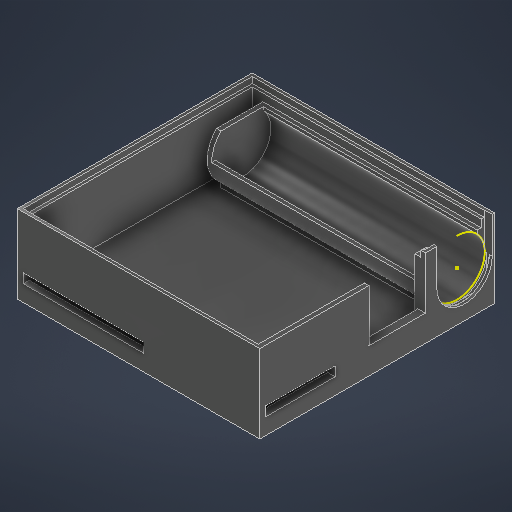
# Autodesk Inventor part: pudelko
Saved by Autodesk Inventor 2026.1 (Build 301233020, 233B)
## iProperties
Created: 2025-08-19
Part Number: pudelko
Material: Generic
Document SubType Name: Modeling
Designer: Paweł
Density: 1 g/cm^3
Appearance: Dark Gray
Mass: 30.7875 g
Surface Area: 279.129 cm^2
Volume: 30.7875 cm^3
Author: Paweł
Autodesk Inventor part; units mm, degrees
ref_plane "YZ Plane" through (0, 0, 0) normal (1, 0, 0) x (0, 1, 0)
ref_plane "XZ Plane" through (0, 0, 0) normal (0, 1, 0) x (-1, 0, 0)
ref_plane "XY Plane" through (0, 0, 0) normal (0, 0, 1) x (1, 0, 0)
sketch "Sketch1" plane through (0, 0, 0) normal (0, 1, 0) x (-1, 0, 0)
  line L0 (77.0121, 67.7143) -> (-2.9879, 67.7143)
  line L1 (-2.9879, 67.7143) -> (-2.9879, -12.2857)
  line L2 (-2.9879, -12.2857) -> (77.0121, -12.2857)
  line L3 (77.0121, -12.2857) -> (77.0121, 67.7143)
  point P0 (0, 0)
  dimension "d0" = 80
  dimension "d1" = 80
  constraints: 8 end point, 2 parallel, 1 horizontal, 1 perpendicular
  measures "d0" distance of L2.end L1.end
  measures "d1" distance of L0.end L1.end
extrude "Extrusion1" add sketch "Sketch1" along normal blind 2
sketch "Sketch2" plane through (0, 2, 0) normal (0, 1, 0) x (1, 0, 0)
  line L0 (2.9879, -67.7143) -> (2.9879, 12.2857) projected
  line L1 (2.9879, 12.2857) -> (-77.0121, 12.2857) projected
  line L2 (-77.0121, 12.2857) -> (-77.0121, -67.7143) projected
  line L3 (-77.0121, -67.7143) -> (2.9879, -67.7143) projected
  line L4 (0.9879, -65.7143) -> (0.9879, 10.2857)
  line L5 (0.9879, 10.2857) -> (-75.0121, 10.2857)
  line L6 (-75.0121, 10.2857) -> (-75.0121, -65.7143)
  line L7 (-75.0121, -65.7143) -> (0.9879, -65.7143)
  point P0 (0, 0)
  dimension "d4" = 2
  constraints: 8 end point, 3 other
  measures "d4" distance between parallel lines of L3 L7
extrude "Extrusion2" add sketch "Sketch2" along normal blind 20
sketch "Sketch4" plane through (-77.0121, 0, 67.7143) normal (0, 0, 1) x (1, 0, 0)
  line L0 (2, 2) -> (2, 22) projected
  line L1 (78, 2) -> (78, 22) projected
  line L2 (2, 12) -> (78, 12)
  line L3 (78, 12) -> (78, 2)
  line L4 (78, 2) -> (2, 2)
  line L5 (2, 2) -> (2, 12)
  line L6 (2, 2) -> (78, 2)
  line L7 (78, 2) -> (78, 7)
  line L8 (78, 7) -> (2, 7)
  line L9 (2, 7) -> (2, 2)
  line L10 (78, 2) -> (62, 2)
  line L11 (62, 2) -> (2, 2)
  line L12 (2, 2) -> (78, 2) projected
  line L13 (2, 2) -> (62, 2)
  line L14 (2, 3.4) -> (78, 3.4)
  line L15 (2, 6.5) -> (78, 6.5)
  line L16 (42, 2) -> (42, 7)
  point P0 (77.0121, 0)
  point P1 (2, 3.4)
  point P2 (42, 3.4)
  point P3 (42, 6.5)
  dimension "d53" = 16
  dimension "d54" = 1.4
  dimension "d55" = 0.5
  dimension "d130" = 40
  constraints: 28 end point, 7 point on line, 5 parallel, 3 perpendicular, 2 collinear, 2 horizontal, 2 midpoint
  measures "d53" distance of L6.end L10.end
  measures "d54" distance between parallel lines of L4 L14
  measures "d55" distance between parallel lines of L8 L15
  measures "d130" distance from line of L14.start L16
extrude "Extrusion4" cut sketch "Sketch4" against normal blind 20 contours L0 L15 L16 L14
sketch "Sketch5" plane through (0.9879, 2, -10.2857) normal (-1, 0, 0) x (0, 0, 1)
  line L0 (76, 0) -> (0, 0) projected
  line L1 (0, 0) -> (0, 20) projected
  circle A0 centre (10, 10) radius 9
  circle A1 centre (10, 10) radius 10
  circle A2 centre (10, 10) radius 10.5
  circle A3 centre (10, 10) radius 9.2
  line L2 (0, 20) -> (76, 20) projected
  line L3 (0, 10) -> (20.5, 10)
  line L4 (13.2016, 0) -> (16.2016, 0)
  line L5 (16.2016, 0) -> (16.2016, 1.5271)
  line L6 (10, 10) -> (10, 20)
  point P0 (10.2857, -2)
  point P1 (78, 0)
  point P2 (10, 0)
  point P3 (13.2016, 0)
  point P4 (13.2016, 20)
  point P5 (6.7984, 20)
  point P6 (0, 13.2016)
  point P7 (0.8, 10)
  point P8 (0, 10)
  point P9 (19.2, 10)
  point P10 (6.7984, 0)
  point P11 (0, 6.7984)
  point P12 (10, 19.2)
  dimension "d11" = 18
  dimension "d12" = 1
  dimension "d13" = 0.5
  dimension "d14" = 0.2
  dimension "d31" = 3
  constraints: 8 end point, 5 point on circle, 4 centre point, 4 midpoint, 4 point on line, 1 horizontal alignment, 1 parallel, 1 perpendicular
  measures "d11" diameter of A0
  measures "d12" radial gap between concentric circles of A0 A1
  measures "d13" radial gap between concentric circles of A1 A2
  measures "d14" radial gap between concentric circles of A0 A3
  measures "d31" distance of L4.start L4.end
extrude "Extrusion5" add sketch "Sketch5" along normal blind 71 contours L0 A2 L5 | L0 A1 L3 A2 | L0 A2 L1 A1 | A1 L3 A3 | L0 L1 A2 | L1 A2 L2 A1 | A1 L6 A3 L3 | L1 L2 A2 picked at (0.4271, 11.4241)
sketch "Sketch10" plane through (0, 2, 0) normal (0, 1, 0) x (1, 0, 0)
  line L0 (-70.0121, -2.9159) -> (-70.0121, -10.2143) projected
  line L1 (-70.0121, 10.2857) -> (-75.0121, 10.2857) projected
  line L2 (-70.0121, -10.2143) -> (-71.5121, -10.2143)
  line L3 (-71.5121, -10.2143) -> (-71.5121, 10.2857)
  line L4 (-71.5121, 10.2857) -> (-70.0121, 10.2857)
  line L5 (-70.0121, 10.2857) -> (-70.0121, -10.2143)
  point P0 (0, 0)
  point P1 (-70.0121, -5.9159)
  dimension "d21" = 1.5
  constraints: 8 end point, 2 parallel, 1 horizontal, 1 perpendicular, 1 point on line
  measures "d21" distance of L3.end L4.end
extrude "Extrusion8" add sketch "Sketch10" along normal up to surface (20 mm away)
sketch "Sketch14" plane through (-70.0121, 2, 10.2143) normal (1, 0, 0) x (0, 0, -1)
  arc A0 (0, 10) -> (4.2984, 1.5271) centre (10.5, 10) ccw projected
  line L0 (0, 0) -> (0, 10) projected
  line L1 (4.2984, 0) -> (0, 0) projected
  line L2 (4.2984, 0) -> (4.2984, 1.5271) projected
  point P0 (10.2143, -2)
extrude "Extrusion11" cut sketch "Sketch14" against normal up to surface (5 mm away)
sketch "Sketch16" plane through (-70.0121, 12, 10.2143) normal (1, 0, 0) x (0, 0, -1)
  arc A0 (1.3, 0) -> (10.5, 9.2) centre (10.5, 0) ccw projected
  arc A1 (0, 0) -> (4.2984, -8.4729) centre (10.5, 0) ccw projected
  circle A2 centre (10.5, 0) radius 10.5
  line L0 (10.5, 10) -> (0, 10) projected
  line L1 (0, 0) -> (0, 10) projected
  point P0 (10.2143, -12)
  point P1 (13.75, -8.6068)
  point P2 (0, 0)
  point P3 (7.2984, 10)
  constraints: 1 centre point, 1 coincident, 1 concentric
extrude "Extrusion13" cut sketch "Sketch16" against normal up to surface (5 mm away) contours L1 L0 A2
sketch "Sketch17" plane through (-77.0121, 0, -12.2857) normal (-1, 0, 0) x (0, 0, 1)
  line L0 (0, 0) -> (0, 22) projected
  line L1 (25.5, 17.7) -> (43, 17.7)
  line L2 (43, 17.7) -> (43, 6.7)
  line L3 (43, 6.7) -> (25.5, 6.7)
  line L4 (25.5, 6.7) -> (25.5, 17.7)
  line L5 (0, 22) -> (80, 22) projected
  line L6 (43, 17.7) -> (43.7211, 17.7)
  line L7 (43.7211, 17.7) -> (43.7211, 6.7)
  line L8 (43.7211, 6.7) -> (43, 6.7)
  line L9 (25.5, 17.7) -> (25, 17.7)
  line L10 (25, 17.7) -> (25, 6.7)
  line L11 (25, 6.7) -> (25.5, 6.7)
  line L12 (25, 17.7) -> (25, 18)
  line L13 (25, 18) -> (43.7211, 18)
  line L14 (43.7211, 18) -> (43.7211, 17.7)
  line L15 (25, 18) -> (25, 22)
  line L16 (43.7211, 18) -> (43.7211, 22)
  point P0 (12.2857, 0)
  point P1 (20.2416, 9.7558)
  point P2 (0, 11)
  dimension "d46" = 11
  dimension "d47" = 17.5
  dimension "d51" = 0.5
  dimension "d52" = 0.3
  dimension "d106" = 4
  constraints: 30 end point, 9 perpendicular, 2 horizontal, 2 parallel, 2 point on line, 1 midpoint, 1 vertical
  measures "d46" distance of L1.end L2.end
  measures "d47" distance of L2.end L3.end
  measures "d51" distance of L1.start L9.end
  measures "d52" distance of L9.end L12.end
  measures "d106" distance between parallel lines of L5 L13
extrude "Extrusion14" cut sketch "Sketch17" against normal blind 4
sketch "Sketch18" plane through (0.9879, 6.5, 65.7143) normal (-1, 0, 0) x (0, 0, 1)
  arc A0 (-66, 14.7) -> (-56.8, 5.5) centre (-66, 5.5) ccw projected
  point P0 (-65.7143, -6.5)
sketch "Sketch19" plane through (-70.0121, 22, -0.2857) normal (0, 0, 1) x (1, 0, 0)
  line L0 (71, 0) -> (71, -0.8) projected
  line L1 (71, 0) -> (0, 0) projected
  line L2 (0, -0.8) -> (0, 0) projected
  line L3 (71, -0.8) -> (0, -0.8) projected
  line L4 (71, -0.8) -> (71, -19.2) projected
  line L5 (0, -0.8) -> (71, -0.8)
  line L6 (71, -0.8) -> (71, -2.5024)
  line L7 (71, -2.5024) -> (0, -2.5024)
  line L8 (0, -2.5024) -> (0, -0.8)
  point P0 (70.0121, -22)
  point P1 (71, -10)
  constraints: 8 end point, 2 parallel, 1 horizontal, 1 perpendicular, 1 point on line
extrude "Extrusion15" cut sketch "Sketch19" against normal blind 13
sketch "Sketch20" plane through (0, 22, 0) normal (0, 1, 0) x (1, 0, 0)
  line L0 (-70.0121, 12.2857) -> (-77.0121, 12.2857) projected
  line L1 (-77.0121, 12.2857) -> (2.9879, 12.2857)
  line L2 (2.9879, 12.2857) -> (2.9879, 10.2857)
  line L3 (2.9879, 10.2857) -> (-77.0121, 10.2857)
  line L4 (-77.0121, 10.2857) -> (-77.0121, 12.2857)
  line L5 (2.9879, -67.7143) -> (2.9879, 12.2857) projected
  point P0 (0, 0)
  point P1 (2.9879, 11.2857)
  dimension "d59" = 2
  constraints: 8 end point, 2 parallel, 1 horizontal, 1 midpoint, 1 perpendicular, 1 point on line
  measures "d59" distance of L3.end L0.end
extrude "Extrusion16" cut sketch "Sketch20" against normal through all
sketch "Sketch22" plane through (0, 2, 0) normal (0, 1, 0) x (1, 0, 0)
  line L0 (-75.0121, -65.7143) -> (-75.0121, 10.2857) projected
  line L1 (-71.5121, -5.9159) -> (-71.5121, 10.2857) projected
  line L2 (-75.0121, 10.2857) -> (-71.5121, 10.2857)
  line L3 (-71.5121, 10.2857) -> (-71.5121, 8.2857)
  line L4 (-71.5121, 8.2857) -> (-75.0121, 8.2857)
  line L5 (-75.0121, 8.2857) -> (-75.0121, 10.2857)
  point P0 (0, 0)
  point P1 (-71.5121, 3.5357)
  dimension "d63" = 2
  constraints: 8 end point, 2 parallel, 1 horizontal, 1 perpendicular, 1 point on line
  measures "d63" distance of L2.end L3.end
extrude "Extrusion17" add sketch "Sketch22" along normal up to surface (20 mm away)
sketch "Sketch25" plane through (-70.0121, 19.4976, -5.6173) normal (0, 1, 0) x (1, 0, 0)
  line L0 (71, 4.6684) -> (0, 4.6684) projected
  line L1 (0, -2.0816) -> (0, 3.8684) projected
  line L2 (71, 4.6684) -> (0, 4.6684)
  line L3 (0, 4.6684) -> (0, 2.6684)
  line L4 (0, 2.6684) -> (71, 2.6684)
  line L5 (71, 2.6684) -> (71, 4.6684)
  point P0 (70.0121, -5.6173)
  point P1 (0, 0)
  point P2 (0, 3.8684)
  point P3 (0, -14.5316)
  dimension "d95" = 2
  constraints: 8 end point, 2 parallel, 1 horizontal, 1 perpendicular, 1 point on line
  measures "d95" distance of L3.end L2.end
extrude "Extrusion20" add sketch "Sketch25" along normal up to surface (2.5024 mm away)
sketch "Sketch26" plane through (0, 22, 0) normal (0, 1, 0) x (1, 0, 0)
  line L0 (-71.5121, 8.2857) -> (-75.0121, 8.2857) projected
  line L1 (-72.6308, 8.2857) -> (-68.2243, 8.2857)
  line L2 (-68.2243, 8.2857) -> (-68.2243, -11.3852)
  line L3 (-68.2243, -11.3852) -> (-72.6308, -11.3852)
  line L4 (-72.6308, -11.3852) -> (-72.6308, 8.2857)
  point P0 (0, 0)
  constraints: 8 end point, 2 parallel, 1 horizontal, 1 perpendicular, 1 point on line
extrude "Extrusion21" cut sketch "Sketch26" against normal up to surface (2.5024 mm away)
sketch "Sketch27" plane through (0.9879, 6.5, 65.7143) normal (-1, 0, 0) x (0, 0, 1)
  arc A0 (-66, 14.7) -> (-56.8, 5.5) centre (-66, 5.5) ccw projected
  circle A1 centre (-66, 5.5) radius 9.2
  point P0 (-65.7143, -6.5)
  point P1 (-56.8, 5.5)
  point P2 (-66, 14.7)
  constraints: 1 centre point, 1 coincident, 1 concentric
extrude "Extrusion22" cut sketch "Sketch27" against normal blind 10
sketch "Sketch28" plane through (0, 22, 0) normal (0, 1, 0) x (1, 0, 0)
  line L0 (2.9879, 9.4857) -> (2.9879, -8.9143) projected
  line L1 (0.9879, 5.6173) -> (-70.0121, 5.6173) projected
  line L2 (-70.0121, -8.9143) -> (-70.0121, 5.6173) projected
  line L3 (0.9879, -8.9143) -> (-70.0121, -8.9143) projected
  line L4 (0.9879, 5.6173) -> (0.9879, -8.9143) projected
  line L5 (2.9879, 9.4857) -> (2.9879, -8.9143) projected
  line L6 (2.9879, 9.4857) -> (0.9879, 9.4857)
  line L7 (0.9879, 9.4857) -> (0.9879, -8.9143)
  line L8 (0.9879, -8.9143) -> (2.9879, -8.9143)
  line L9 (2.9879, -8.9143) -> (2.9879, 9.4857)
  point P0 (0, 0)
  point P1 (2.9879, -8.9143)
  constraints: 8 end point, 2 parallel, 1 horizontal, 1 perpendicular
extrude "Extrusion23" cut sketch "Sketch28" against normal blind 10 contours L0 L8 L4 L7 L6
sketch "Sketch29" plane through (0.9879, 22, -8.2857) normal (1, 0, 0) x (0, 0, -1)
  arc A0 (1.2, -10) -> (-2.6684, -2.5024) centre (-8, -10) ccw projected
  line L0 (-1.2985, -3.6969) -> (-1.3342, -2.5024)
  line L1 (-2.6684, -2.5024) -> (0, -2.5024) projected
  arc A1 (1.2, -10) -> (-2.6684, -2.5024) centre (-8, -10) ccw projected
  line L2 (1.2, 0) -> (1.2, -10) projected
  line L3 (0, 0) -> (1.2, 0) projected
  line L4 (0, 0) -> (0, -2.5024) projected
  line L5 (-2.6684, -2.5024) -> (0, -2.5024) projected
  point P0 (-8.2857, -22)
  constraints: 2 end point, 1 midpoint, 1 point on circle
extrude "Extrusion24" cut sketch "Sketch29" against normal up to surface (71 mm away) contours A0 L1 L0
sketch "Sketch30" plane through (0, 22, 0) normal (0, 1, 0) x (1, 0, 0)
  line L0 (-77.0121, 10.2857) -> (-77.0121, -12.7143) projected
  line L1 (2.9879, 10.2857) -> (-77.0121, 10.2857) projected
  line L2 (-77.0121, -31.4354) -> (-77.0121, -67.7143) projected
  line L3 (-77.0121, -67.7143) -> (2.9879, -67.7143) projected
  line L4 (0.9879, -65.7143) -> (-75.0121, -65.7143) projected
  line L5 (-75.0121, -65.7143) -> (-75.0121, -31.4354) projected
  line L6 (-75.0121, -12.7143) -> (-75.0121, -31.4354) projected
  line L7 (-75.0121, -12.7143) -> (-75.0121, 8.2857) projected
  line L8 (0.9879, 8.2857) -> (-75.0121, 8.2857) projected
  line L9 (0.9879, 9.2857) -> (-76.0121, 9.2857)
  line L10 (-76.0121, 9.2857) -> (-76.0121, -12.7143)
  line L11 (-76.0121, -12.7143) -> (-76.0121, -31.4354)
  line L12 (-76.0121, -31.4354) -> (-76.0121, -66.7143)
  line L13 (-76.0121, -66.7143) -> (0.9879, -66.7143)
  line L14 (-48.0121, -67.7143) -> (-48.0121, -65.7143)
  line L15 (-48.0121, -65.7143) -> (-48.0121, 10.2857)
  line L16 (2.9879, -8.9143) -> (0.9879, -8.9143) projected
  line L17 (0.9879, -8.9143) -> (0.9879, -65.7143) projected
  line L18 (0.9879, -65.7143) -> (-75.0121, -65.7143) projected
  line L19 (-75.0121, -65.7143) -> (-75.0121, -31.4354) projected
  line L20 (-75.0121, -31.4354) -> (-77.0121, -31.4354) projected
  line L21 (-77.0121, -31.4354) -> (-77.0121, -67.7143) projected
  line L22 (-77.0121, -67.7143) -> (2.9879, -67.7143) projected
  line L23 (2.9879, -67.7143) -> (2.9879, -8.9143) projected
  line L24 (0.9879, -66.7143) -> (1.9879, -66.7143)
  line L25 (1.9879, -66.7143) -> (1.9879, -8.9143)
  line L26 (0.9879, 8.2857) -> (0.9879, 9.4857) projected
  line L27 (0.9879, 9.4857) -> (2.9879, 9.4857) projected
  line L28 (2.9879, 9.4857) -> (2.9879, 10.2857) projected
  line L29 (-77.0121, 10.2857) -> (2.9879, 10.2857) projected
  line L30 (-77.0121, 10.2857) -> (-77.0121, -12.7143) projected
  line L31 (-77.0121, -12.7143) -> (-75.0121, -12.7143) projected
  line L32 (-75.0121, -12.7143) -> (-75.0121, 8.2857) projected
  line L33 (0.9879, 8.2857) -> (-75.0121, 8.2857) projected
  point P0 (0, 0)
  point P1 (2.9879, -67.7143)
  dimension "d107" = 1
  dimension "d108" = 29
  constraints: 18 end point, 3 perpendicular, 3 point on line, 1 midpoint, 4 other
  measures "d107" distance between parallel lines of L8 L9
  measures "d108" distance between parallel lines of L2 L14
extrude "Extrusion25" add sketch "Sketch30" along normal blind 2 contours L1 L15 L9 L10 L31 L0 | L1 L28 L27 L26 L9 L15 | L10 L9 L15 L8 L7 L31 | L9 L26 L8 L15 | L12 L13 L14 L3 L2 L20 | L13 L24 L25 L16 L23 L3 L14
sketch "Sketch31" plane through (2.9879, 0, 67.7143) normal (1, 0, 0) x (0, 0, -1)
  arc A0 (58.8, 12) -> (77.2, 12) centre (68, 12) ccw projected
  line L0 (58.8, 2.8) -> (77.2, 2.8)
  line L1 (0, 0) -> (78, 0) projected
  line L2 (58.8, 12) -> (58.8, 0)
  line L3 (77.2, 0) -> (77.2, 12)
  point P0 (67.7143, 0)
  point P1 (68, 2.8)
  constraints: 6 end point, 4 point on line, 2 perpendicular, 1 parallel, 1 tangent
extrude "Extrusion26" cut sketch "Sketch31" against normal blind 2 contours A0 L0 L2 | A0 L3 L0
sketch "Sketch32" plane through (2.9879, 2.8, 8.9143) normal (0, 1, 0) x (1, 0, 0)
  line L0 (-2, 9.2) -> (-2, 18.4) projected
  line L1 (-2, 18.4) -> (-2, 15.9015) projected
  line L2 (-2, 15.9015) -> (-73, 15.9015) projected
  line L3 (-73, 0) -> (-73, 15.9015) projected
  line L4 (-2, 0) -> (-73, 0) projected
  line L5 (-2, 0) -> (-2, 9.2) projected
  line L6 (0, -58.8) -> (0, 19.2) projected
  line L7 (0, 18.4) -> (-2, 18.4) projected
  line L8 (0, 0) -> (-0.5, 0)
  line L9 (-0.5, 0) -> (-0.5, 18.4)
  line L10 (-0.5, 18.4) -> (0, 18.4)
  line L11 (0, 18.4) -> (0, 0)
  line L12 (-2, 0) -> (-1.3662, 0)
  line L13 (-1.3662, 0) -> (-1.3662, 18.7503)
  line L14 (-1.3662, 18.7503) -> (-2, 18.7503)
  line L15 (-2, 18.7503) -> (-2, 0)
  point P0 (-2.9879, 8.9143)
  point P1 (-1.3662, 18.4)
  dimension "d113" = 0.5
  constraints: 16 end point, 4 parallel, 2 horizontal, 2 perpendicular, 2 point on line
  measures "d113" distance of L9.end L10.end
extrude "Extrusion27" add sketch "Sketch32" along normal up to surface contours L0 L7 L13 L12 L5 | L8 L9 L7 L6 round surface about axis through (0.9879, 12, -0.2857) along (-1, 0, 0) radius 9.2 far side no
sketch "Sketch34" plane through (2.9879, 0, -10.2857) normal (0, 0, -1) x (-1, 0, 0)
  point P0 (2.9879, 0)
sketch "Sketch35" plane through (0, 24, 0) normal (0, 1, 0) x (1, 0, 0)
  line L0 (-77.0121, -12.7143) -> (-75.0121, -12.7143) projected
  line L1 (-76.0121, -12.7143) -> (-76.0121, 9.2857)
  line L2 (1.9879, -66.7143) -> (-76.0121, -66.7143) projected
  line L3 (-77.0121, -12.7143) -> (-75.0121, -12.7143) projected
  line L4 (2.9879, -67.7143) -> (2.9879, 10.2857) projected
  line L5 (-75.0121, 8.2857) -> (0.9879, 8.2857) projected
  line L6 (0.9879, 8.2857) -> (0.9879, 9.4857) projected
  line L7 (0.9879, 9.4857) -> (2.9879, 9.4857) projected
  line L8 (2.9879, 9.4857) -> (2.9879, 10.2857) projected
  line L9 (2.9879, 10.2857) -> (-77.0121, 10.2857) projected
  line L10 (-77.0121, 10.2857) -> (-77.0121, -12.7143) projected
  line L11 (-77.0121, -12.7143) -> (-75.0121, -12.7143) projected
  line L12 (-75.0121, -12.7143) -> (-75.0121, 8.2857) projected
  line L13 (-76.0121, 9.2857) -> (0.9879, 9.2857)
  point P0 (0, 0)
  point P1 (-76.0121, -12.7143)
  dimension "d117" = 76
  constraints: 4 end point, 2 midpoint, 1 perpendicular, 1 point on line, 1 vertical, 1 vertical alignment
  measures "d117" distance from line of L2 L1.end
extrude "Extrusion28" cut sketch "Sketch35" against normal blind 2 contours L1 L13 L6 L5 L12 L0
sketch "Sketch36" plane through (0.9879, 12, 8.9143) normal (0, 0, -1) x (-1, 0, 0)
  line L0 (-1.5, 0) -> (-2, 0) projected
  line L1 (-1.5, 0) -> (-1.5, -9.2) projected
  line L2 (-1.5, -9.2) -> (-0.6338, -9.2) projected
  line L3 (-0.6338, -9.2) -> (-0.6338, 0) projected
  line L4 (0, 0) -> (-0.6338, 0) projected
  line L5 (0, 10) -> (0, 0) projected
  line L6 (-1, 10) -> (0, 10) projected
  line L7 (-1, 10) -> (-1, 12) projected
  line L8 (-2, 12) -> (-1, 12) projected
  line L9 (-2, 0) -> (-2, 12) projected
  line L10 (-0.6338, 0) -> (-0.6338, 10)
  line L11 (-1.5, 0) -> (-1.5, 12)
  point P0 (0.9879, -12)
  constraints: 4 end point, 1 midpoint, 1 perpendicular, 1 point on line
extrude "Extrusion29" cut sketch "Sketch36" against normal blind 3 contours L11 L8 L7 L6 L10 L3 L2 L1
sketch "Sketch37" plane through (0, 22, 0) normal (0, 1, 0) x (1, 0, 0)
  line L0 (1.9879, -11.9143) -> (1.6217, -11.9143) projected
  line L1 (1.6217, -11.9143) -> (1.6217, -8.9143) projected
  line L2 (1.6217, -8.9143) -> (0.9879, -8.9143) projected
  line L3 (0.9879, -8.9143) -> (0.9879, -65.7143) projected
  line L4 (0.9879, -65.7143) -> (-75.0121, -65.7143) projected
  line L5 (-75.0121, -65.7143) -> (-75.0121, -31.4354) projected
  line L6 (-75.0121, -31.4354) -> (-76.0121, -31.4354) projected
  line L7 (-76.0121, -31.4354) -> (-76.0121, -66.7143) projected
  line L8 (-76.0121, -66.7143) -> (1.9879, -66.7143) projected
  line L9 (1.9879, -66.7143) -> (1.9879, -11.9143) projected
  line L10 (-76.0121, -66.7143) -> (1.9879, -66.7143) projected
  line L11 (-76.0121, -31.4354) -> (-76.0121, -66.7143) projected
  line L12 (-27.0121, -66.7143) -> (-27.0121, -65.7143)
  line L13 (0.9879, -65.7143) -> (-75.0121, -65.7143) projected
  line L14 (0.9879, -38.2143) -> (1.9879, -38.2143)
  line L15 (0.9879, -65.7143) -> (0.9879, -5.9159) projected
  point P0 (0, 0)
  point P1 (-27.0121, -65.7143)
  point P2 (-75.0121, -38.2143)
  dimension "d134" = 29
  dimension "d135" = 28.5
  constraints: 6 point on line, 4 end point, 2 perpendicular
  measures "d134" distance between parallel lines of L12 L9
  measures "d135" distance between parallel lines of L8 L14
extrude "Extrusion30" cut sketch "Sketch37" against normal blind 4 contours L9 L8 L12 L4 L3 L14
sketch "Sketch38" plane through (0, 0, 0) normal (0, -1, 0) x (1, 0, 0)
  line L0 (-77.0121, -10.2857) -> (2.9879, -10.2857) projected
  line L1 (2.9879, 67.7143) -> (2.9879, -10.2857) projected
  line L2 (-77.0121, 67.7143) -> (2.9879, 67.7143) projected
  line L3 (-77.0121, -10.2857) -> (-77.0121, 67.7143) projected
  point P0 (0, 0)
extrude "Extrusion31" add sketch "Sketch38" along normal blind 2
sketch "Sketch39" plane through (2.9879, 24, 67.7143) normal (1, 0, 0) x (0, 0, -1)
  line L0 (0, -17.5) -> (0, -20.6) projected
  line L1 (0, -17.5) -> (25, -17.5)
  line L2 (2, -22) -> (2, -6) projected
  line L3 (0, -20.6) -> (25, -20.6)
  line L4 (25, -17.5) -> (25, -20.6)
  point P0 (67.7143, -24)
  point P1 (2, -2)
  point P2 (2, -17.5)
  point P3 (2, -20.6)
  dimension "d131" = 25
  constraints: 7 end point, 2 horizontal, 1 vertical
  measures "d131" distance of L0.start L1.end
extrude "Extrusion32" cut sketch "Sketch39" against normal up to surface (2 mm away) contours L1 L4 L3 L2
sketch "Sketch40" plane through (0, 24, 0) normal (0, 1, 0) x (1, 0, 0)
  line L0 (0.9879, -38.2143) -> (1.9879, -38.2143) projected
  line L1 (1.9879, -38.2143) -> (1.9879, -11.9143) projected
  line L2 (1.9879, -11.9143) -> (1.6217, -11.9143) projected
  line L3 (1.6217, -11.9143) -> (1.6217, -8.9143) projected
  line L4 (1.6217, -8.9143) -> (0.9879, -8.9143) projected
  line L5 (0.9879, -8.9143) -> (0.9879, -38.2143) projected
  line L6 (2.4879, -11.9143) -> (1.9879, -11.9143) projected
  line L7 (1.9879, -11.9143) -> (1.9879, -66.7143) projected
  line L8 (1.9879, -66.7143) -> (-76.0121, -66.7143) projected
  line L9 (-76.0121, -66.7143) -> (-76.0121, -31.4354) projected
  line L10 (-76.0121, -31.4354) -> (-77.0121, -31.4354) projected
  line L11 (-77.0121, -31.4354) -> (-77.0121, -67.7143) projected
  line L12 (-77.0121, -67.7143) -> (2.9879, -67.7143) projected
  line L13 (2.9879, -67.7143) -> (2.9879, -8.9143) projected
  line L14 (2.9879, -8.9143) -> (2.4879, -8.9143) projected
  line L15 (2.4879, -8.9143) -> (2.4879, -11.9143) projected
  line L16 (0.9879, -31.4354) -> (2.9879, -31.4354)
  line L17 (0.9879, -12.7143) -> (2.9879, -12.7143)
  point P0 (0, 0)
  point P1 (-77.0121, -12.7143)
  constraints: 4 end point, 4 point on line, 2 horizontal alignment, 2 perpendicular
extrude "Extrusion33" cut sketch "Sketch40" against normal blind 17.3 contours L5 L17 L1 L16 | L1 L17 L13 L16
sketch "Sketch42" plane through (-75.0121, 6.7, 31.4354) normal (0, 0, -1) x (-1, 0, 0)
  line L0 (0, 0) -> (0, 15.3) projected
  line L1 (2, 0) -> (0, 0) projected
  line L2 (2, 17.3) -> (2, 0) projected
  line L3 (1, 17.3) -> (2, 17.3) projected
  line L4 (1, 15.3) -> (1, 17.3) projected
  line L5 (0, 15.3) -> (1, 15.3) projected
  point P0 (-75.0121, -6.7)
extrude "Extrusion34" add sketch "Sketch42" along normal up to surface (18.7211 mm away)
sketch "Sketch43" plane through (0.9879, 2, 5.9159) normal (-1, 0, 0) x (0, 0, 1)
  line L0 (25.5195, 20) -> (25.5195, 4.7) projected
  line L1 (25.5195, 4.7) -> (6.7984, 4.7) projected
  line L2 (6.7984, 4.7) -> (6.7984, 20) projected
  line L3 (2.9984, 20) -> (6.7984, 20) projected
  line L4 (2.9984, 20) -> (2.9984, 10) projected
  line L5 (2.9984, 10) -> (4.2984, 10) projected
  arc A0 (0, 1.5271) -> (4.2984, 10) centre (-6.2016, 10) ccw projected
  line L6 (0, 1.5271) -> (0, 0) projected
  line L7 (59.7984, 0) -> (0, 0) projected
  line L8 (59.7984, 0) -> (59.7984, 1.4) projected
  line L9 (59.7984, 1.4) -> (36.7984, 1.4) projected
  line L10 (36.7984, 1.4) -> (36.7984, 4.5) projected
  line L11 (36.7984, 4.5) -> (59.7984, 4.5) projected
  line L12 (59.7984, 4.5) -> (59.7984, 16) projected
  line L13 (59.7984, 16) -> (32.2984, 16) projected
  line L14 (32.2984, 16) -> (32.2984, 20) projected
  line L15 (25.5195, 20) -> (32.2984, 20) projected
  line L16 (6.7984, 4.7) -> (6.7984, -0.1103)
  line L17 (59.7984, 0) -> (0, 0) projected
  point P0 (-5.9159, -2)
  point P1 (6.7984, 0)
  constraints: 2 end point, 1 perpendicular
extrude "Extrusion35" add sketch "Sketch43" along normal blind 1 contours L16 L7 L6 A0 L5 L4 L3 L2
sketch "Sketch44" plane through (2.9879, 12, -9.4857) normal (1, 0, 0) x (0, 0, -1)
  line L0 (-40.9211, -5.3) -> (-40.9211, 12) projected
  line L1 (-77.2, 12) -> (-40.9211, 12) projected
  line L2 (-77.2, 12) -> (-77.2, -14) projected
  line L3 (0.8, -14) -> (-77.2, -14) projected
  line L4 (0.8, 12) -> (0.8, -14) projected
  line L5 (0, 12) -> (0.8, 12) projected
  line L6 (0, 12) -> (0, 0) projected
  arc A0 (-18.4, 0) -> (0, 0) centre (-9.2, 0) ccw projected
  line L7 (-18.4, 0) -> (-18.4, 12) projected
  line L8 (-22.2, 12) -> (-18.4, 12) projected
  line L9 (-22.2, 12) -> (-22.2, -5.3) projected
  line L10 (-22.2, -5.3) -> (-40.9211, -5.3) projected
  line L11 (-52.2, -5.5) -> (-52.2, -8.6) projected
  line L12 (-52.2, -8.6) -> (-75.2, -8.6) projected
  line L13 (-75.2, -8.6) -> (-75.2, -5.5) projected
  line L14 (-75.2, -5.5) -> (-52.2, -5.5) projected
  point P0 (-9.4857, -12)
extrude "Extrusion36" add sketch "Sketch44" along normal blind 0.5
body "Solid1"
